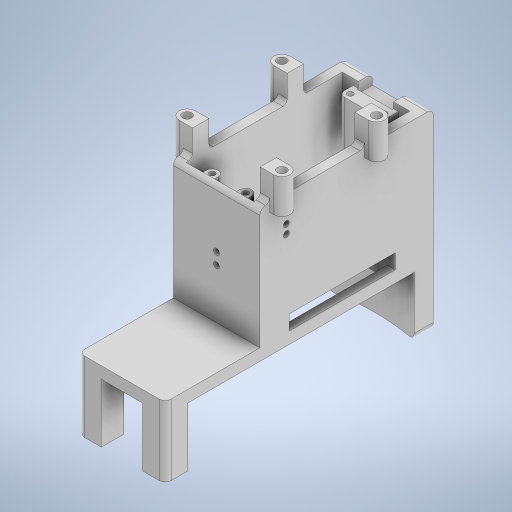
# Autodesk Inventor part: base
Saved by Autodesk Inventor 2023 (Build 270158000, 158)
## iProperties
Created: 2023-01-28
Part Number: base
Material: 一般
Document SubType Name: Modeling
Designer: taka2
Density: 1 g/cm^3
Appearance: 既定
Author: taka2
Autodesk Inventor part; units mm, degrees
ref_plane "YZ Plane" through (0, 0, 0) normal (1, 0, 0) x (0, 1, 0)
ref_plane "XZ Plane" through (0, 0, 0) normal (0, 1, 0) x (-1, 0, 0)
ref_plane "XY Plane" through (0, 0, 0) normal (0, 0, 1) x (1, 0, 0)
sketch "スケッチ1" plane through (0, 0, 0) normal (0, 1, 0) x (-1, 0, 0)
  line L0 (14.7, 0) -> (-14.7, 0)
  line L1 (-14.7, 0) -> (-14.7, -91.2)
  line L2 (-14.7, -91.2) -> (14.7, -91.2)
  line L3 (14.7, -91.2) -> (14.7, 0)
  line L4 (0, 0) -> (0, -124.5084)
  line L5 (14.7, -7.7) -> (7, -7.7)
  line L6 (7, -7.7) -> (7, 0)
  line L7 (-7, 0) -> (-7, -7.7)
  line L8 (-7, -7.7) -> (-14.7, -7.7)
  arc A0 (-14.7, -84.7) -> (14.7, -84.7) centre (0, -13.42) ccw
  line L9 (-12, -78.2) -> (12, -78.2)
  line L10 (12, -78.2) -> (12, -42.2)
  line L11 (12, -42.2) -> (-12, -42.2)
  line L12 (-12, -42.2) -> (-12, -78.2)
  line L13 (14.7, -60.2) -> (-14.7, -60.2)
  point P0 (0, -86.2)
  point P1 (0, -91.2)
  dimension "d0" = 29.4
  dimension "d3" = 14
  dimension "d4" = 5
  dimension "d5" = 1.5
  dimension "d6" = 78.5
  dimension "d8" = 36
  dimension "d9" = 24
  dimension "d108" = 26
  constraints: 28 end point, 10 point on line, 5 parallel, 4 horizontal, 4 perpendicular, 3 point on circle, 2 midpoint, 1 centre point, 1 symmetric about line, 1 vertical, 5 other
  measures "d0" distance of L0.start L0.end
  measures "d3" distance between parallel lines of L7 L6
  measures "d4" distance of point (0, -86.2) point (0, -91.2)
  measures "d5" vertical distance of A0.start point (0, -86.2)
  measures "d6" vertical distance of L7.end point (0, -86.2)
  measures "d8" distance of L11.end L9.start
  measures "d9" distance between parallel lines of L12 L10
  measures "d108" vertical distance of L13.start point (0, -86.2)
extrude "押し出し1" add sketch "スケッチ1" against normal blind 20 contours L3 L5 L6 L0 | L7 L8 L1 L0 | L3 L2 L4 A0 | L4 L2 L1 A0
extrude "押し出し2" add sketch "スケッチ1" along normal blind 4 contours L3 L5 L6 L0 | L6 L5 L3 L13 L10 L11 L4 L0 | L4 L11 L12 L13 L1 L8 L7 L0 | L3 A0 L4 L9 L10 L13 | L7 L8 L1 L0 | L3 L2 L4 A0 | A0 L1 L13 L12 L9 L4 | L4 L2 L1 A0
sketch "スケッチ2" plane through (0, 4, 0) normal (0, 1, 0) x (1, 0, 0)
  line L0 (-14.7, 91.2) -> (14.7, 91.2) projected
  line L1 (-14.7, 91.2) -> (14.7, 91.2)
  line L2 (14.7, 91.2) -> (14.7, 78.2)
  line L3 (14.7, 78.2) -> (-14.7, 78.2)
  line L4 (-14.7, 78.2) -> (-14.7, 91.2)
  line L5 (14.7, 0) -> (14.7, 91.2) projected
  line L6 (-14.7, 91.2) -> (-14.7, 0) projected
  line L7 (14.7, 32.2) -> (-14.7, 32.2)
  line L8 (-14.7, 32.2) -> (-14.7, 42.2)
  line L9 (-14.7, 42.2) -> (14.7, 42.2)
  line L10 (14.7, 42.2) -> (14.7, 32.2)
  point P0 (0, 0)
  point P1 (12, 42.2)
  point P2 (14.7, 42.2)
  point P3 (12, 78.2)
  dimension "d15" = 10
  constraints: 16 end point, 5 point on line, 4 parallel, 2 horizontal, 2 perpendicular
  measures "d15" distance of L7.end L8.end
extrude "押し出し3" add sketch "スケッチ2" along normal blind 5 contours L0 L2 L3 L4 | L9 L5 L7 L6
sketch "スケッチ3" plane through (0, 9, 0) normal (0, 1, 0) x (1, 0, 0)
  line L0 (-14.7, 91.2) -> (14.7, 91.2) projected
  line L1 (14.7, 91.2) -> (-14.7, 91.2)
  line L2 (-14.7, 91.2) -> (-14.7, 32.2)
  line L3 (-14.7, 32.2) -> (14.7, 32.2)
  line L4 (14.7, 32.2) -> (14.7, 91.2)
  arc A0 (2.8, 54.6123) -> (-2.8, 54.6123) centre (0, 60.2) ccw
  line L5 (-12, 42.2) -> (-12, 78.2) projected
  line L6 (-12, 60.2) -> (12, 60.2)
  line L7 (12, 78.2) -> (12, 42.2) projected
  line L8 (0, 91.2) -> (0, 32.2)
  line L9 (6.25, 70.95) -> (-6.25, 70.95)
  line L10 (-6.25, 70.95) -> (-6.25, 38.95)
  line L11 (-6.25, 38.95) -> (6.25, 38.95)
  line L12 (6.25, 38.95) -> (6.25, 70.95)
  line L13 (-6.25, 66.45) -> (6.25, 66.45)
  line L14 (-6.25, 43.45) -> (6.25, 43.45)
  arc A1 (-2.8, 53.45) -> (2.8, 53.45) centre (0, 53.45) ccw
  line L15 (-2.8, 53.45) -> (-2.8, 54.6123)
  line L16 (2.8, 53.45) -> (2.8, 54.6123)
  circle A2 centre (0, 68.7) radius 1
  circle A3 centre (0, 41.2) radius 1
  point P0 (0, 0)
  dimension "d18" = 12.5
  dimension "d19" = 4.5
  dimension "d20" = 4.5
  dimension "d21" = 2.8
  dimension "d22" = 13
  dimension "d23" = 2
  dimension "d24" = 2.25
  dimension "d25" = 2.25
  dimension "d26" = 23
  constraints: 28 end point, 9 point on line, 5 midpoint, 5 parallel, 4 centre point, 4 perpendicular, 4 point on circle, 2 horizontal, 2 tangent, 1 coincident, 1 equal radius, 1 vertical, 1 other
  measures "d18" distance of L9.start L9.end
  measures "d19" distance of L13.end L9.start
  measures "d20" distance of L11.end L14.end
  measures "d21" radius of A1
  measures "d22" distance from line of A1.centre L13
  measures "d23" diameter of A2
  measures "d24" distance from line of L13 A2.centre
  measures "d25" distance from line of L11 A3.centre
  measures "d26" distance of L14.start L13.start
extrude "押し出し4" add sketch "スケッチ3" along normal blind 4 contours L0 L8 L9 L10 L11 L3 L2 | L0 L4 L3 L8 L11 L12 L9 | L9 L12 L13 L8 A2 | L8 A2 L13 L10 L9 | L11 L10 L14 L8 A3 | L8 A3 L14 L12 L11 | L12 A0 L13 | L13 A0 L10 | L12 L14 L8 A1 L16 A0 | A0 L15 A1 L8 L14 L10
extrude "押し出し5" add sketch "スケッチ3" along normal blind 8 contours L9 L12 L13 L8 A2 | L8 A2 L13 L10 L9 | L11 L10 L14 L8 A3 | L8 A3 L14 L12 L11
sketch "スケッチ7" plane through (0, 13, 0) normal (0, 1, 0) x (1, 0, 0)
  line L0 (-14.7, 32.2) -> (14.7, 32.2) projected
  line L1 (0, 32.2) -> (0, 91.2)
  line L2 (-14.7, 91.2) -> (14.7, 91.2) projected
  line L3 (-14.7, 91.2) -> (14.7, 91.2)
  line L4 (14.7, 91.2) -> (14.7, 32.2)
  line L5 (14.7, 32.2) -> (-14.7, 32.2)
  line L6 (-14.7, 32.2) -> (-14.7, 91.2)
  line L7 (11.5, 86.4) -> (-11.5, 86.4)
  line L8 (-11.5, 86.4) -> (-11.5, 33.4)
  line L9 (-11.5, 33.4) -> (11.5, 33.4)
  line L10 (11.5, 33.4) -> (11.5, 86.4)
  circle A0 centre (-5.7, 36.4) radius 1
  circle A1 centre (5.7, 36.4) radius 1
  line L11 (-14.7, 84.7) -> (-14.7, 7.7) projected
  line L12 (-14.7, 59.9) -> (14.7, 59.9)
  arc A2 (-3.7, 36.4) -> (-7.7, 36.4) centre (-5.7, 36.4) ccw
  line L13 (-7.7, 36.4) -> (-7.7, 33.4)
  line L14 (-3.7, 36.4) -> (-3.7, 33.4)
  arc A3 (7.7, 36.4) -> (3.7, 36.4) centre (5.7, 36.4) ccw
  line L15 (7.7, 36.4) -> (7.7, 33.4)
  line L16 (3.7, 36.4) -> (3.7, 33.4)
  circle A4 centre (-5.7, 83.4) radius 1
  circle A5 centre (5.7, 83.4) radius 1
  arc A6 (-7.7, 83.4) -> (-5.7, 81.4) centre (-5.7, 83.4) ccw
  line L17 (-7.7, 83.4) -> (-7.7, 86.4)
  line L18 (7.7, 83.4) -> (7.7, 86.4)
  arc A7 (5.7, 81.4) -> (7.7, 83.4) centre (5.7, 83.4) ccw
  line L19 (-5.7, 81.4) -> (5.7, 81.4)
  point P0 (0, 0)
  point P1 (-3.7, 83.4)
  dimension "d49" = 1.2
  dimension "d50" = 23
  dimension "d51" = 53
  dimension "d52" = 11.4
  dimension "d53" = 2
  dimension "d54" = 3
  dimension "d55" = 26.5
  dimension "d56" = 4
  constraints: 34 end point, 14 symmetric about line, 8 centre point, 8 point on circle, 5 perpendicular, 4 parallel, 4 point on line, 4 tangent, 2 coincident, 2 horizontal, 2 midpoint, 7 other
  measures "d49" distance between parallel lines of L0 L9
  measures "d50" distance between parallel lines of L10 L8
  measures "d51" distance between parallel lines of L9 L7
  measures "d52" distance of A1.centre A0.centre
  measures "d53" diameter of A1
  measures "d54" distance from line of L9 A1.centre
  measures "d55" vertical distance of L8.end L12.start
  measures "d56" distance between parallel lines of L14 L13
extrude "押し出し11" add sketch "スケッチ7" along normal blind 30 contours L9 L13 A2 L14 | L16 A3 L15 L9 | L19 A6 L17 L7 L1 | L1 L7 L18 A7 L19 | A0 | A1 | A4 | A5
extrude "押し出し12" add sketch "スケッチ7" along normal blind 32 contours L6 L12 L8 L9 L1 L0 | L1 L9 L10 L12 L4 L0 | L6 L2 L1 L7 L8 L12 | L12 L10 L7 L1 L2 L4
sketch "スケッチ8" plane through (0, 43, 0) normal (0, 1, 0) x (1, 0, 0)
  circle A0 centre (-5.7, 83.4) radius 1
  circle A1 centre (5.7, 83.4) radius 1
  circle A2 centre (-5.7, 36.4) radius 1
  circle A3 centre (5.7, 36.4) radius 1
  arc A4 (5.7, 81.4) -> (7.7, 83.4) centre (5.7, 83.4) ccw projected
  arc A5 (-7.7, 83.4) -> (-5.7, 81.4) centre (-5.7, 83.4) ccw projected
  arc A6 (-3.7, 36.4) -> (-7.7, 36.4) centre (-5.7, 36.4) ccw projected
  arc A7 (7.7, 36.4) -> (3.7, 36.4) centre (5.7, 36.4) ccw projected
  point P0 (0, 0)
  dimension "d61" = 2
  constraints: 4 centre point, 4 concentric, 3 equal radius
  measures "d61" diameter of A1
extrude "押し出し13" cut sketch "スケッチ8" against normal blind 10
sketch "スケッチ9" plane through (0, 45, 0) normal (0, 1, 0) x (1, 0, 0)
  line L0 (-14.7, 91.2) -> (14.7, 91.2) projected
  line L1 (-6, 91.2) -> (6, 91.2)
  line L2 (6, 91.2) -> (6, 85.9)
  line L3 (6, 85.9) -> (-6, 85.9)
  line L4 (-6, 85.9) -> (-6, 91.2)
  line L5 (0, 91.2) -> (0, 32.2)
  line L6 (14.7, 32.2) -> (-14.7, 32.2) projected
  point P0 (0, 0)
  dimension "d64" = 12
  dimension "d65" = 5.3
  constraints: 10 end point, 2 midpoint, 2 parallel, 1 horizontal, 1 perpendicular, 1 point on line, 1 other
  measures "d64" distance between parallel lines of L4 L2
  measures "d65" distance of L1.end L2.end
extrude "押し出し14" cut sketch "スケッチ9" against normal blind 3.5
sketch "スケッチ11" plane through (0, 45, 0) normal (0, 1, 0) x (1, 0, 0)
  line L0 (-14.7, 91.2) -> (14.7, 91.2) projected
  line L1 (0, 91.2) -> (0, 32.2)
  line L2 (-14.7, 32.2) -> (14.7, 32.2) projected
  circle A0 centre (-16.1, 38.3) radius 1.55
  circle A1 centre (-16.1, 70.5) radius 1.55
  circle A2 centre (16.1, 38.3) radius 1.55
  circle A3 centre (16.1, 70.5) radius 1.55
  line L3 (-16.1, 70.5) -> (-16.1, 38.3)
  arc A4 (-16.1, 73.25) -> (-16.1, 67.75) centre (-16.1, 70.5) ccw
  line L4 (-16.1, 73.25) -> (-11.5, 73.25)
  line L5 (-11.5, 33.4) -> (-11.5, 86.4) projected
  line L6 (-16.1, 67.75) -> (-11.5, 67.75)
  line L7 (-11.5, 41.05) -> (-16.1, 41.05)
  line L8 (-11.5, 35.55) -> (-16.1, 35.55)
  arc A5 (-16.1, 41.05) -> (-16.1, 35.55) centre (-16.1, 38.3) ccw
  line L9 (16.1, 70.5) -> (16.1, 38.3)
  arc A6 (16.1, 67.75) -> (16.1, 73.25) centre (16.1, 70.5) ccw
  line L10 (16.1, 73.25) -> (11.5, 73.25)
  line L11 (16.1, 67.75) -> (11.5, 67.75)
  line L12 (11.5, 41.05) -> (16.1, 41.05)
  line L13 (11.5, 35.55) -> (16.1, 35.55)
  arc A7 (16.1, 35.55) -> (16.1, 41.05) centre (16.1, 38.3) ccw
  line L14 (11.5, 35.55) -> (11.5, 41.05)
  line L15 (12, 78.2) -> (12, 42.2) projected
  line L16 (11.5, 67.75) -> (11.5, 73.25)
  point P0 (0, 0)
  dimension "d72" = 32.2
  dimension "d73" = 32.2
  dimension "d74" = 6.1
  dimension "d75" = 3.1
  dimension "d76" = 2.75
  constraints: 26 end point, 14 symmetric about line, 8 centre point, 8 point on circle, 8 point on line, 4 coincident, 4 tangent, 3 horizontal, 2 equal radius, 2 midpoint, 2 parallel, 1 collinear, 1 vertical, 4 other
  measures "d72" distance of A3.centre L3.start
  measures "d73" distance of L3.start L3.end
  measures "d74" vertical distance of L2.start L3.end
  measures "d75" diameter of A1
  measures "d76" radius of A4
extrude "押し出し16" add sketch "スケッチ11" along normal blind 9 and the other way blind 2.75 contours A0 | A1 | A2 | A3 | A4 L4 L5 L6 | L7 L5 L8 A5 | L11 L15 L10 A6 | L11 L16 L10 L15 | L12 A7 L13 L14
sketch "スケッチ12" plane through (0, 54, 0) normal (0, 1, 0) x (1, 0, 0)
  circle A0 centre (-16.1, 70.5) radius 1.55
  circle A1 centre (-16.1, 38.3) radius 1.55
  circle A2 centre (16.1, 38.3) radius 1.55
  circle A3 centre (16.1, 70.5) radius 1.55
  arc A4 (-16.1, 73.25) -> (-16.1, 67.75) centre (-16.1, 70.5) ccw projected
  arc A5 (-16.1, 41.05) -> (-16.1, 35.55) centre (-16.1, 38.3) ccw projected
  arc A6 (16.1, 35.55) -> (16.1, 41.05) centre (16.1, 38.3) ccw projected
  arc A7 (16.1, 67.75) -> (16.1, 73.25) centre (16.1, 70.5) ccw projected
  point P0 (0, 0)
  dimension "d80" = 3.1
  constraints: 4 centre point, 4 concentric, 3 equal radius
  measures "d80" diameter of A3
extrude "押し出し17" cut sketch "スケッチ12" against normal blind 6.5
sketch "スケッチ17" plane through (-14.7, 4, -32.2) normal (0, 0, 1) x (1, 0, 0)
  line L0 (0, 41) -> (29.4, 41) projected
  line L1 (14.7, 41) -> (14.7, -4)
  circle A0 centre (14.7, 21) radius 1
  circle A1 centre (14.7, 17) radius 1
  dimension "d127" = 2
  dimension "d128" = 4
  dimension "d129" = 20
  constraints: 2 centre point, 2 end point, 2 midpoint, 2 point on line, 1 equal radius, 1 vertical
  measures "d127" diameter of A0
  measures "d128" distance of A1.centre A0.centre
  measures "d129" distance of A0.centre point (14.7, 41)
extrude "押し出し22" cut sketch "スケッチ17" against normal up to surface (1.2 mm away)
fillet "フィレット7" radius 2 3 edges at (0, 45, -32.2) (-10.35, 45, -91.2) (10.35, 45, -91.2)
fillet "フィレット8" radius 2 2 edges at (-14.7, -8, 0) (14.7, -8, 0)
fillet "フィレット6" radius 1.5 8 edges at (-13.1, 45, -35.55) (13.1, 45, -35.55) (-13.1, 45, -67.75) (13.1, 45, -67.75) (-13.1, 45, -41.05) (13.1, 45, -41.05) (13.1, 45, -73.25) (-13.1, 45, -73.25)
fillet "フィレット9" radius 2 2 edges at (14.7, -20, -87.95) (-14.7, -20, -87.95)
sketch "スケッチ18" plane through (14.7, 0, -7.7) normal (1, 0, 0) x (0, 0, -1)
  line L0 (33.5, 45) -> (33.5, 9)
  line L1 (24.5, 4) -> (24.5, 43) projected
  line L2 (34.85, 45) -> (58.55, 45) projected
  line L3 (34.5, 9) -> (70.5, 9) projected
  circle A0 centre (33.5, 36) radius 1
  circle A1 centre (33.5, 33) radius 1
  point P0 (-7.7, 0)
  dimension "d133" = 9
  dimension "d134" = 2
  dimension "d135" = 9
  dimension "d136" = 3
  constraints: 4 point on line, 2 centre point, 2 end point, 1 equal radius, 1 vertical
  measures "d133" distance between parallel lines of L1 L0
  measures "d134" diameter of A0
  measures "d135" distance of A0.centre L0.start
  measures "d136" distance of A1.centre A0.centre
extrude "押し出し23" cut sketch "スケッチ18" against normal up to surface (3.2 mm away)
